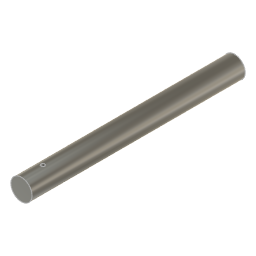
Guide Bar (Autodesk Fusion 360 design; units mm, degrees)
Autodesk Fusion 360 part; units mm, degrees
cylinder "CylinderPrimitive1" add diameter 12.7 height 127 placed x (1, 0, 0) y (0, 1, 0) z (0, 0, 1) at (0, 0, 0)
move_body "Move1" bodies 1 to x (1, 0, 0) y (0, 0, -1) z (0, 1, 0) at (0, -127, 9.1022)
sketch "Sketch4" plane through (0, 0, 0) normal (1, 0, 0) x (0, 1, 0)
  circle A0 centre (-114.3, 9.1022) radius 1.1049
  point P0 (-127, 9.1022)
  dimension "d8" = 2.2098
  dimension "d9" = 12.7
  measures "d8" diameter of A0
  measures "d9" distance of P0 A0.centre
extrude "Extrude1" cut sketch "Sketch4" along normal mid plane 50.8
move_body "Move2" bodies 1 to x (0, 0, -1) y (0, 1, 0) z (1, 0, 0) at (-9.1022, 0, 9.1022)
thread "Thread1" [suppressed]
hole "Hole1" [suppressed]
thread "Thread2" [suppressed]
